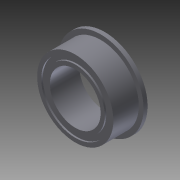
# Autodesk Inventor part: bearing_1.125OD
Saved by Autodesk Inventor 2012 (Build 160160000, 160)
## iProperties
Created: 2011-01-09
Part Number: bearing_1.125OD
Material: Steel
Document SubType Name: Modeling
Designer: Antonella Wilby
Mass: 58.0147 g
Surface Area: 28.819 cm^2
Volume: 7.39041 cm^3
Density: 7.85 g/cm^3
Author: Antonella Wilby
Autodesk Inventor part; units mm, degrees
ref_plane "YZ Plane" through (0, 0, 0) normal (1, 0, 0) x (0, 1, 0)
ref_plane "XZ Plane" through (0, 0, 0) normal (0, 1, 0) x (-1, 0, 0)
ref_plane "XY Plane" through (0, 0, 0) normal (0, 0, 1) x (1, 0, 0)
sketch "Sketch1" plane through (0, 0, 0) normal (0, 0, 1) x (1, 0, 0)
  line L0 (-7.5032, 0) -> (7.5032, 0) projected
  line L1 (0, -7.5032) -> (0, 7.5032) projected
  circle A0 centre (0, 0) radius 5.3594
  circle A1 centre (0, 0) radius 3.175
  dimension "d0" = 6.35
  dimension "d1" = 10.7188
  constraints: 2 centre point, 2 coincident
  measures "d0" diameter of A1
  measures "d1" diameter of A0
extrude "Base" add sketch "Sketch1" along normal mid plane 3.683 contours A1 L1 A0 L0 | L0 A0 L1 A1 | A1 L0 A0 L1 | L1 A0 L0 A1
sketch "Sketch2" plane through (0, 0, 1.8415) normal (0, 0, 1) x (1, 0, 0)
  circle A0 centre (0, 0) radius 5.3594 projected
  circle A1 centre (0, 0) radius 4.7625
  dimension "d4" = 9.525
  constraints: 1 centre point, 1 coincident
  measures "d4" diameter of A1
extrude "Flange Cutaway" cut sketch "Sketch2" against normal blind 3.175
sketch "Sketch3" plane through (0, 0, 1.8415) normal (0, 0, 1) x (1, 0, 0)
  circle A0 centre (0, 0) radius 3.175 projected
  circle A1 centre (0, 0) radius 4.7625 projected
  circle A2 centre (0, 0) radius 3.683
  circle A3 centre (0, 0) radius 4.2545
  dimension "d11" = 0.508
  dimension "d12" = 0.508
  constraints: 2 centre point, 2 coincident
  measures "d11" radial gap between concentric circles of A1 A3
  measures "d12" radial gap between concentric circles of A2 A0
extrude "Cutaway" cut sketch "Sketch3" against normal blind 0.1984 contours A3
mirror "Mirror1" about plane through (0, 0, 0) normal (0, 0, 1) of "Cutaway"
body "Solid1"
